Autodesk Fusion 360 part; units mm, degrees
note: some values were not read from the file. Chosen so that the rebuilt part matches the saved one: which face or edge a step refers to. Set by a fixed rule: which sketch regions a step uses.
(part 4 of 4)
sketch "Fingers Bottom" plane through (0, 0, 0) normal (0, 0, 1) x (1, 0, 0) in component "Bottom"
  arc A0 (-85.6137, -27.905) -> (-84, -26.7758) centre (-84.7071, -27.4829) ccw
  arc A1 (-84, -119.2242) -> (-85.6137, -118.095) centre (-84.7071, -118.5171) ccw
  arc A2 (-84, -39.2242) -> (-85.6137, -38.095) centre (-84.7071, -38.5171) ccw
  line L0 (-84, -26.7758) -> (-84, -19.2242)
  arc A3 (-85.6137, -107.905) -> (-84, -106.7758) centre (-84.7071, -107.4829) ccw
  arc A4 (-87.175, -126.7758) -> (-85.5613, -127.905) centre (-86.4679, -127.4829) ccw
  arc A5 (-84, -139.2242) -> (-85.6137, -138.095) centre (-84.7071, -138.5171) ccw
  line L1 (-84, -146.7758) -> (-84, -139.2242)
  line L2 (-85.5613, -107.905) -> (-85.6137, -107.905)
  arc A6 (-87.175, -146.7758) -> (-85.5613, -147.905) centre (-86.4679, -147.4829) ccw
  line L3 (-85.5613, -147.905) -> (-85.6137, -147.905)
  arc A7 (-87.175, -26.7758) -> (-85.5613, -27.905) centre (-86.4679, -27.4829) ccw
  line L4 (-87.175, -119.2242) -> (-87.175, -126.7758)
  line L5 (-85.5613, -127.905) -> (-85.6137, -127.905)
  arc A8 (-85.5613, -18.095) -> (-87.175, -19.2242) centre (-86.4679, -18.5171) ccw
  line L6 (-85.6137, -38.095) -> (-85.5613, -38.095)
  arc A9 (-87.175, -106.7758) -> (-85.5613, -107.905) centre (-86.4679, -107.4829) ccw
  line L7 (-85.6137, -18.095) -> (-85.5613, -18.095)
  line L8 (-85.5613, -27.905) -> (-85.6137, -27.905)
  arc A10 (-85.6137, -127.905) -> (-84, -126.7758) centre (-84.7071, -127.4829) ccw
  line L9 (-85.6137, -118.095) -> (-85.5613, -118.095)
  line L10 (-84, -46.7758) -> (-84, -39.2242)
  arc A11 (-84, -79.2242) -> (-85.6137, -78.095) centre (-84.7071, -78.5171) ccw
  arc A12 (-84, -59.2242) -> (-85.6137, -58.095) centre (-84.7071, -58.5171) ccw
  arc A13 (-85.5613, -58.095) -> (-87.175, -59.2242) centre (-86.4679, -58.5171) ccw
  arc A14 (-87.175, -86.7758) -> (-85.5613, -87.905) centre (-86.4679, -87.4829) ccw
  line L11 (-87.175, -59.2242) -> (-87.175, -66.7758)
  line L12 (0, 0) -> (-240, 0) construction
  line L13 (-85.5613, -47.905) -> (-85.6137, -47.905)
  arc A15 (-87.175, -66.7758) -> (-85.5613, -67.905) centre (-86.4679, -67.4829) ccw
  arc A16 (-87.175, -46.7758) -> (-85.5613, -47.905) centre (-86.4679, -47.4829) ccw
  line L14 (-85.6137, -78.095) -> (-85.5613, -78.095)
  line L15 (-84, -66.7758) -> (-84, -59.2242)
  arc A17 (-85.6137, -47.905) -> (-84, -46.7758) centre (-84.7071, -47.4829) ccw
  line L16 (-87.175, -139.2242) -> (-87.175, -146.7758)
  line L17 (-85.6137, -138.095) -> (-85.5613, -138.095)
  line L18 (-84, -126.7758) -> (-84, -119.2242)
  line L19 (-87.175, -39.2242) -> (-87.175, -46.7758)
  line L20 (-85.6137, -58.095) -> (-85.5613, -58.095)
  arc A18 (-85.6137, -147.905) -> (-84, -146.7758) centre (-84.7071, -147.4829) ccw
  arc A19 (-85.5613, -118.095) -> (-87.175, -119.2242) centre (-86.4679, -118.5171) ccw
  arc A20 (-85.5613, -78.095) -> (-87.175, -79.2242) centre (-86.4679, -78.5171) ccw
  line L21 (-87.175, -99.2242) -> (-87.175, -106.7758)
  arc A21 (-85.5613, -138.095) -> (-87.175, -139.2242) centre (-86.4679, -138.5171) ccw
  line L22 (-87.175, -79.2242) -> (-87.175, -86.7758)
  arc A22 (-84, -99.2242) -> (-85.6137, -98.095) centre (-84.7071, -98.5171) ccw
  line L23 (0, 0) -> (0, -184) construction
  arc A23 (-85.5613, -98.095) -> (-87.175, -99.2242) centre (-86.4679, -98.5171) ccw
  line L24 (-84, -86.7758) -> (-84, -79.2242)
  line L25 (-85.6137, -98.095) -> (-85.5613, -98.095)
  line L26 (-85.5613, -87.905) -> (-85.6137, -87.905)
  arc A24 (-85.6137, -87.905) -> (-84, -86.7758) centre (-84.7071, -87.4829) ccw
  line L27 (0, -184) -> (-240, -184) construction
  line L28 (-240, 0) -> (-240, -184) construction
  line L29 (-85.5613, -67.905) -> (-85.6137, -67.905)
  arc A25 (-85.6137, -67.905) -> (-84, -66.7758) centre (-84.7071, -67.4829) ccw
  arc A26 (-85.5613, -158.095) -> (-87.175, -159.2242) centre (-86.4679, -158.5171) ccw
  arc A27 (-84, -19.2242) -> (-85.6137, -18.095) centre (-84.7071, -18.5171) ccw
  line L30 (-87.175, -19.2242) -> (-87.175, -26.7758)
  arc A28 (-85.6137, -167.905) -> (-84, -166.7758) centre (-84.7071, -167.4829) ccw
  line L31 (-85.6137, -158.095) -> (-85.5613, -158.095)
  line L32 (-84, -166.7758) -> (-84, -159.2242)
  arc A29 (-87.175, -166.7758) -> (-85.5613, -167.905) centre (-86.4679, -167.4829) ccw
  arc A30 (-85.5613, -38.095) -> (-87.175, -39.2242) centre (-86.4679, -38.5171) ccw
  line L33 (-85.5613, -167.905) -> (-85.6137, -167.905)
  line L34 (-87.175, -159.2242) -> (-87.175, -166.7758)
  arc A31 (-84, -159.2242) -> (-85.6137, -158.095) centre (-84.7071, -158.5171) ccw
  line L35 (-84, -106.7758) -> (-84, -99.2242)
  line L36 (-240, -2) -> (0, -2)
  point P0 (0, -184)
  dimension "d1377" = 20
  dimension "d1378" = 20
  dimension "d1379" = 2
  dimension "d1380" = 0.4221
  dimension "d1381" = 9.81
  dimension "d1382" = 2
  dimension "d1383" = 16.095
  dimension "d1384" = 3.175
  dimension "d1385" = 2
  dimension "d1386" = 2
  dimension "d1387" = 0.4221
  dimension "d1388" = 0.4221
  dimension "d1389" = 0.7071
  dimension "d1390" = 0.7071
  dimension "d1391" = 0.7071
  dimension "d1392" = 84
  dimension "d1393" = 0.4221
  dimension "d1395" = 240
  dimension "d1622" = 182
  constraint horizontal L27
  constraint perpendicular L32 L33
  constraint vertical A28.centre A31.centre
  constraint perpendicular L12 L23
  constraint perpendicular L27 L28
  constraint coincident P0 L23.end
  constraint coincident L12.start L23.start
  measures "d1379" diameter of A31
  measures "d1380" distance of A31.centre L31
  measures "d1381" distance of L31 L33
  measures "d1382" diameter of A28
  measures "d1383" distance of L27 L33
  measures "d1384" distance of L32 L34
  measures "d1385" diameter of A26
  measures "d1386" diameter of A29
  measures "d1387" distance of A26.centre L31
  measures "d1388" distance of A29.centre L33
  measures "d1389" distance of A29.centre L34
  measures "d1390" distance of A28.centre L32
  measures "d1391" distance of A26.centre L34
  measures "d1392" distance of L23 L32
  measures "d1393" distance of A28.centre L33
  measures "d1395" distance of L27.end P0
  measures "d1622" distance of L27 L36
sketch "Fingers" plane through (0, 0, 0) normal (0, 0, 1) x (1, 0, 0) in component "Top"
  arc A0 (-85.6137, 16.095) -> (-84, 17.2242) centre (-84.7071, 16.5171) ccw
  arc A1 (-85.6137, 36.095) -> (-84, 37.2242) centre (-84.7071, 36.5171) ccw
  line L0 (-87.175, 44.7758) -> (-87.175, 37.2242)
  arc A2 (-84, 24.7758) -> (-85.6137, 25.905) centre (-84.7071, 25.4829) ccw
  line L1 (-87.175, 24.7758) -> (-87.175, 17.2242)
  line L2 (-87.175, 64.7758) -> (-87.175, 57.2242)
  line L3 (-85.6137, 125.905) -> (-85.5613, 125.905)
  arc A3 (-84, 144.7758) -> (-85.6137, 145.905) centre (-84.7071, 145.4829) ccw
  arc A4 (-85.6137, 156.095) -> (-84, 157.2242) centre (-84.7071, 156.5171) ccw
  arc A5 (-85.5613, 125.905) -> (-87.175, 124.7758) centre (-86.4679, 125.4829) ccw
  line L4 (-87.175, 144.7758) -> (-87.175, 137.2242)
  line L5 (-87.175, 164.7758) -> (-87.175, 157.2242)
  line L6 (-87.175, 104.7758) -> (-87.175, 97.2242)
  line L7 (-85.6137, 145.905) -> (-85.5613, 145.905)
  arc A6 (-85.5613, 105.905) -> (-87.175, 104.7758) centre (-86.4679, 105.4829) ccw
  line L8 (-85.5613, 96.095) -> (-85.6137, 96.095)
  arc A7 (-84, 124.7758) -> (-85.6137, 125.905) centre (-84.7071, 125.4829) ccw
  arc A8 (-87.175, 137.2242) -> (-85.5613, 136.095) centre (-86.4679, 136.5171) ccw
  line L9 (-85.5613, 116.095) -> (-85.6137, 116.095)
  arc A9 (-84, 84.7758) -> (-85.6137, 85.905) centre (-84.7071, 85.4829) ccw
  line L10 (-84, 157.2242) -> (-84, 164.7758)
  line L11 (-85.5613, 156.095) -> (-85.6137, 156.095)
  line L12 (-84, 137.2242) -> (-84, 144.7758)
  arc A10 (-85.6137, 116.095) -> (-84, 117.2242) centre (-84.7071, 116.5171) ccw
  line L13 (-85.6137, 165.905) -> (-85.5613, 165.905)
  arc A11 (-84, 164.7758) -> (-85.6137, 165.905) centre (-84.7071, 165.4829) ccw
  arc A12 (-87.175, 157.2242) -> (-85.5613, 156.095) centre (-86.4679, 156.5171) ccw
  arc A13 (-85.5613, 165.905) -> (-87.175, 164.7758) centre (-86.4679, 165.4829) ccw
  line L14 (-85.6137, 85.905) -> (-85.5613, 85.905)
  arc A14 (-87.175, 117.2242) -> (-85.5613, 116.095) centre (-86.4679, 116.5171) ccw
  arc A15 (-85.6137, 96.095) -> (-84, 97.2242) centre (-84.7071, 96.5171) ccw
  arc A16 (-85.5613, 145.905) -> (-87.175, 144.7758) centre (-86.4679, 145.4829) ccw
  arc A17 (-85.5613, 85.905) -> (-87.175, 84.7758) centre (-86.4679, 85.4829) ccw
  arc A18 (-87.175, 97.2242) -> (-85.5613, 96.095) centre (-86.4679, 96.5171) ccw
  arc A19 (-87.175, 37.2242) -> (-85.5613, 36.095) centre (-86.4679, 36.5171) ccw
  arc A20 (-84, 44.7758) -> (-85.6137, 45.905) centre (-84.7071, 45.4829) ccw
  line L15 (0, 0) -> (-240, 0) construction
  line L16 (-85.5613, 16.095) -> (-85.6137, 16.095)
  arc A21 (-85.5613, 25.905) -> (-87.175, 24.7758) centre (-86.4679, 25.4829) ccw
  line L17 (-85.6137, 65.905) -> (-85.5613, 65.905)
  line L18 (-84, 37.2242) -> (-84, 44.7758)
  line L19 (-85.6137, 45.905) -> (-85.5613, 45.905)
  arc A22 (-87.175, 17.2242) -> (-85.5613, 16.095) centre (-86.4679, 16.5171) ccw
  arc A23 (-87.175, 57.2242) -> (-85.5613, 56.095) centre (-86.4679, 56.5171) ccw
  line L20 (-85.5613, 36.095) -> (-85.6137, 36.095)
  arc A24 (-84, 64.7758) -> (-85.6137, 65.905) centre (-84.7071, 65.4829) ccw
  line L21 (0, 182) -> (-240, 182) construction
  arc A25 (-85.5613, 45.905) -> (-87.175, 44.7758) centre (-86.4679, 45.4829) ccw
  arc A26 (-85.5613, 65.905) -> (-87.175, 64.7758) centre (-86.4679, 65.4829) ccw
  line L22 (-87.175, 84.7758) -> (-87.175, 77.2242)
  line L23 (-84, 57.2242) -> (-84, 64.7758)
  arc A27 (-85.6137, 136.095) -> (-84, 137.2242) centre (-84.7071, 136.5171) ccw
  line L24 (-84, 17.2242) -> (-84, 24.7758)
  line L25 (-85.6137, 25.905) -> (-85.5613, 25.905)
  arc A28 (-85.6137, 56.095) -> (-84, 57.2242) centre (-84.7071, 56.5171) ccw
  line L26 (-240, 182) -> (-240, 0) construction
  line L27 (0, 182) -> (0, 0) construction
  line L28 (-85.5613, 56.095) -> (-85.6137, 56.095)
  line L29 (-84, 77.2242) -> (-84, 84.7758)
  line L30 (-84, 117.2242) -> (-84, 124.7758)
  arc A29 (-87.175, 77.2242) -> (-85.5613, 76.095) centre (-86.4679, 76.5171) ccw
  line L31 (-85.6137, 105.905) -> (-85.5613, 105.905)
  arc A30 (-84, 104.7758) -> (-85.6137, 105.905) centre (-84.7071, 105.4829) ccw
  line L32 (-84, 97.2242) -> (-84, 104.7758)
  line L33 (-87.175, 124.7758) -> (-87.175, 117.2242)
  line L34 (-85.5613, 76.095) -> (-85.6137, 76.095)
  arc A31 (-85.6137, 76.095) -> (-84, 77.2242) centre (-84.7071, 76.5171) ccw
  line L35 (-85.5613, 136.095) -> (-85.6137, 136.095)
  dimension "d1479" = 20
  dimension "d1480" = 20
  dimension "d1481" = 2
  dimension "d1482" = 0.4221
  dimension "d1483" = 9.81
  dimension "d1484" = 2
  dimension "d1485" = 16.095
  dimension "d1486" = 3.175
  dimension "d1487" = 2
  dimension "d1488" = 2
  dimension "d1489" = 0.4221
  dimension "d1490" = 0.4221
  dimension "d1491" = 0.7071
  dimension "d1492" = 0.7071
  dimension "d1493" = 0.7071
  dimension "d1494" = 84
  dimension "d1495" = 0.4221
  dimension "d1496" = 182
  dimension "d1497" = 240
  constraint horizontal L15
  constraint perpendicular L16 L24
  constraint vertical A2.centre A0.centre
  constraint perpendicular L21 L27
  constraint perpendicular L15 L26
  constraint coincident L15.start L27.end
  measures "d1481" diameter of A2
  measures "d1482" distance of A2.centre L25
  measures "d1483" distance of L16 L25
  measures "d1484" diameter of A0
  measures "d1485" distance of L15 L16
  measures "d1486" distance of L1 L24
  measures "d1487" diameter of A21
  measures "d1488" diameter of A22
  measures "d1489" distance of A21.centre L25
  measures "d1490" distance of A22.centre L16
  measures "d1491" distance of A22.centre L1
  measures "d1492" distance of A0.centre L24
  measures "d1493" distance of A21.centre L1
  measures "d1494" distance of L24 L27
  measures "d1495" distance of A0.centre L16
  measures "d1496" distance of L15.start L21.start
  measures "d1497" distance of L15.end L15.start
sketch "Projection" plane through (0, 0, 0) normal (0, 0, 1) x (1, 0, 0) in component "Brace"
  line L0 (3.175, 14.7758) -> (3.175, 0)
  line L1 (3.175, 0) -> (15.095, 0)
  line L2 (15.095, 0) -> (15.095, 1.5613)
  arc A0 (16.2242, 3.175) -> (15.095, 1.5613) centre (15.5171, 2.4679) ccw
  line L3 (16.2242, 3.175) -> (23.7758, 3.175)
  arc A1 (24.905, 1.5613) -> (23.7758, 3.175) centre (24.4829, 2.4679) ccw
  line L4 (24.905, 1.5613) -> (24.905, 0)
  line L5 (24.905, 0) -> (35.095, 0)
  line L6 (35.095, 0) -> (35.095, 1.5613)
  arc A2 (36.2242, 3.175) -> (35.095, 1.5613) centre (35.5171, 2.4679) ccw
  line L7 (36.2242, 3.175) -> (43.7758, 3.175)
  arc A3 (44.905, 1.5613) -> (43.7758, 3.175) centre (44.4829, 2.4679) ccw
  line L8 (44.905, 1.5613) -> (44.905, 0)
  line L9 (44.905, 0) -> (56.825, 0)
  line L10 (56.825, 0) -> (56.825, 14.7758)
  arc A4 (58.4387, 15.905) -> (56.825, 14.7758) centre (57.5321, 15.4829) ccw
  line L11 (58.4387, 15.905) -> (60, 15.905)
  line L12 (60, 15.905) -> (60, 26.095)
  line L13 (60, 26.095) -> (58.4387, 26.095)
  arc A5 (56.825, 27.2242) -> (58.4387, 26.095) centre (57.5321, 26.5171) ccw
  line L14 (56.825, 27.2242) -> (56.825, 34.7758)
  arc A6 (58.4387, 35.905) -> (56.825, 34.7758) centre (57.5321, 35.4829) ccw
  line L15 (58.4387, 35.905) -> (60, 35.905)
  line L16 (60, 35.905) -> (60, 46.095)
  line L17 (60, 46.095) -> (58.4387, 46.095)
  arc A7 (56.825, 47.2242) -> (58.4387, 46.095) centre (57.5321, 46.5171) ccw
  line L18 (56.825, 47.2242) -> (56.825, 54.7758)
  arc A8 (58.4387, 55.905) -> (56.825, 54.7758) centre (57.5321, 55.4829) ccw
  line L19 (58.4387, 55.905) -> (60, 55.905)
  line L20 (60, 55.905) -> (60, 66.095)
  line L21 (60, 66.095) -> (58.4387, 66.095)
  arc A9 (56.825, 67.2242) -> (58.4387, 66.095) centre (57.5321, 66.5171) ccw
  line L22 (56.825, 67.2242) -> (56.825, 74.7758)
  arc A10 (58.4387, 75.905) -> (56.825, 74.7758) centre (57.5321, 75.4829) ccw
  line L23 (58.4387, 75.905) -> (60, 75.905)
  line L24 (60, 75.905) -> (60, 86.095)
  line L25 (60, 86.095) -> (58.4387, 86.095)
  arc A11 (56.825, 87.2242) -> (58.4387, 86.095) centre (57.5321, 86.5171) ccw
  line L26 (56.825, 87.2242) -> (56.825, 94.7758)
  arc A12 (58.4387, 95.905) -> (56.825, 94.7758) centre (57.5321, 95.4829) ccw
  line L27 (58.4387, 95.905) -> (60, 95.905)
  line L28 (60, 95.905) -> (60, 106.095)
  line L29 (60, 106.095) -> (58.4387, 106.095)
  arc A13 (56.825, 107.2242) -> (58.4387, 106.095) centre (57.5321, 106.5171) ccw
  line L30 (56.825, 107.2242) -> (56.825, 114.7758)
  arc A14 (58.4387, 115.905) -> (56.825, 114.7758) centre (57.5321, 115.4829) ccw
  line L31 (58.4387, 115.905) -> (60, 115.905)
  line L32 (60, 115.905) -> (60, 126.095)
  line L33 (60, 126.095) -> (58.4387, 126.095)
  arc A15 (56.825, 127.2242) -> (58.4387, 126.095) centre (57.5321, 126.5171) ccw
  line L34 (56.825, 127.2242) -> (56.825, 134.7758)
  arc A16 (58.4387, 135.905) -> (56.825, 134.7758) centre (57.5321, 135.4829) ccw
  line L35 (58.4387, 135.905) -> (60, 135.905)
  line L36 (60, 135.905) -> (60, 146.095)
  line L37 (60, 146.095) -> (58.4387, 146.095)
  arc A17 (56.825, 147.2242) -> (58.4387, 146.095) centre (57.5321, 146.5171) ccw
  line L38 (56.825, 147.2242) -> (56.825, 154.7758)
  arc A18 (58.4387, 155.905) -> (56.825, 154.7758) centre (57.5321, 155.4829) ccw
  line L39 (58.4387, 155.905) -> (60, 155.905)
  line L40 (60, 155.905) -> (60, 166.095)
  line L41 (60, 166.095) -> (58.4387, 166.095)
  arc A19 (56.825, 167.2242) -> (58.4387, 166.095) centre (57.5321, 166.5171) ccw
  line L42 (56.825, 167.2242) -> (56.825, 182)
  line L43 (56.825, 182) -> (44.905, 182)
  line L44 (44.905, 182) -> (44.905, 180.4387)
  arc A20 (43.7758, 178.825) -> (44.905, 180.4387) centre (44.4829, 179.5321) ccw
  line L45 (43.7758, 178.825) -> (36.2242, 178.825)
  arc A21 (35.095, 180.4387) -> (36.2242, 178.825) centre (35.5171, 179.5321) ccw
  line L46 (35.095, 180.4387) -> (35.095, 182)
  line L47 (35.095, 182) -> (24.905, 182)
  line L48 (24.905, 182) -> (24.905, 180.4387)
  arc A22 (23.7758, 178.825) -> (24.905, 180.4387) centre (24.4829, 179.5321) ccw
  line L49 (23.7758, 178.825) -> (16.2242, 178.825)
  arc A23 (15.095, 180.4387) -> (16.2242, 178.825) centre (15.5171, 179.5321) ccw
  line L50 (15.095, 180.4387) -> (15.095, 182)
  line L51 (15.095, 182) -> (3.175, 182)
  line L52 (3.175, 182) -> (3.175, 167.2242)
  arc A24 (1.5613, 166.095) -> (3.175, 167.2242) centre (2.4679, 166.5171) ccw
  line L53 (1.5613, 166.095) -> (0, 166.095)
  line L54 (0, 166.095) -> (0, 155.905)
  line L55 (0, 155.905) -> (1.5613, 155.905)
  arc A25 (3.175, 154.7758) -> (1.5613, 155.905) centre (2.4679, 155.4829) ccw
  line L56 (3.175, 154.7758) -> (3.175, 147.2242)
  arc A26 (1.5613, 146.095) -> (3.175, 147.2242) centre (2.4679, 146.5171) ccw
  line L57 (1.5613, 146.095) -> (0, 146.095)
  line L58 (0, 146.095) -> (0, 135.905)
  line L59 (0, 135.905) -> (1.5613, 135.905)
  arc A27 (3.175, 134.7758) -> (1.5613, 135.905) centre (2.4679, 135.4829) ccw
  line L60 (3.175, 134.7758) -> (3.175, 127.2242)
  arc A28 (1.5613, 126.095) -> (3.175, 127.2242) centre (2.4679, 126.5171) ccw
  line L61 (1.5613, 126.095) -> (0, 126.095)
  line L62 (0, 126.095) -> (0, 115.905)
  line L63 (0, 115.905) -> (1.5613, 115.905)
  arc A29 (3.175, 114.7758) -> (1.5613, 115.905) centre (2.4679, 115.4829) ccw
  line L64 (3.175, 114.7758) -> (3.175, 107.2242)
  arc A30 (1.5613, 106.095) -> (3.175, 107.2242) centre (2.4679, 106.5171) ccw
  line L65 (1.5613, 106.095) -> (0, 106.095)
  line L66 (0, 106.095) -> (0, 95.905)
  line L67 (0, 95.905) -> (1.5613, 95.905)
  arc A31 (3.175, 94.7758) -> (1.5613, 95.905) centre (2.4679, 95.4829) ccw
  line L68 (3.175, 94.7758) -> (3.175, 87.2242)
  arc A32 (1.5613, 86.095) -> (3.175, 87.2242) centre (2.4679, 86.5171) ccw
  line L69 (1.5613, 86.095) -> (0, 86.095)
  line L70 (0, 86.095) -> (0, 75.905)
  line L71 (0, 75.905) -> (1.5613, 75.905)
  arc A33 (3.175, 74.7758) -> (1.5613, 75.905) centre (2.4679, 75.4829) ccw
  line L72 (3.175, 74.7758) -> (3.175, 67.2242)
  arc A34 (1.5613, 66.095) -> (3.175, 67.2242) centre (2.4679, 66.5171) ccw
  line L73 (1.5613, 66.095) -> (0, 66.095)
  line L74 (0, 66.095) -> (0, 55.905)
  line L75 (0, 55.905) -> (1.5613, 55.905)
  arc A35 (3.175, 54.7758) -> (1.5613, 55.905) centre (2.4679, 55.4829) ccw
  line L76 (3.175, 54.7758) -> (3.175, 47.2242)
  arc A36 (1.5613, 46.095) -> (3.175, 47.2242) centre (2.4679, 46.5171) ccw
  line L77 (1.5613, 46.095) -> (0, 46.095)
  line L78 (0, 46.095) -> (0, 35.905)
  line L79 (0, 35.905) -> (1.5613, 35.905)
  arc A37 (3.175, 34.7758) -> (1.5613, 35.905) centre (2.4679, 35.4829) ccw
  line L80 (3.175, 34.7758) -> (3.175, 27.2242)
  arc A38 (1.5613, 26.095) -> (3.175, 27.2242) centre (2.4679, 26.5171) ccw
  line L81 (1.5613, 26.095) -> (0, 26.095)
  line L82 (0, 26.095) -> (0, 15.905)
  line L83 (0, 15.905) -> (1.5613, 15.905)
  arc A39 (3.175, 14.7758) -> (1.5613, 15.905) centre (2.4679, 15.4829) ccw
sketch "pHSUpport" plane through (0, 0, 0) normal (0, 0, 1) x (1, 0, 0)
  line L0 (-126.3121, 423.4789) -> (-0.0021, 423.4789)
  line L1 (-0.0021, 423.4789) -> (-0.0021, 307.4298)
  line L2 (-63.1571, 307.4298) -> (-126.3121, 307.4298)
  line L3 (-126.3121, 307.4298) -> (-126.3121, 423.4789)
  circle A0 centre (-95.0428, 331.8598) radius 15
  line L4 (-63.1571, 307.4298) -> (-63.1571, 368.1283)
  line L5 (-63.1571, 368.1283) -> (-0.0021, 368.1283)
  dimension "d1660" = 30
  constraint horizontal L0
  constraint vertical L1
  constraint horizontal L2
  constraint vertical L3
  constraint perpendicular L2 L4
  constraint coincident L1 L5.end
  constraint perpendicular L1 L5
  measures "d1660" diameter of A0
sketch "Sketch1" plane through (0, 0, 0) normal (0, 0, 1) x (1, 0, 0) in component "Peristaltic Pump Support"
  circle A0 centre (53.5964, 47.8456) radius 1.5
  circle A1 centre (22.5964, 47.8456) radius 1.5
  line L0 (55.0964, 58.3456) -> (55.0964, 6.3456) construction
  circle A2 centre (38.0964, 32.3456) radius 15
  line L1 (21.0964, 58.3456) -> (55.0964, 58.3456) construction
  circle A3 centre (38.0964, 56.8456) radius 1.5
  line L2 (55.0964, 6.3456) -> (21.0964, 6.3456) construction
  circle A4 centre (22.5964, 16.8456) radius 1.5
  line L3 (21.0964, 6.3456) -> (21.0964, 58.3456) construction
  circle A5 centre (53.5964, 16.8456) radius 1.5
  circle A6 centre (38.0964, 7.8456) radius 1.5
  point P0 (38.0964, 6.3456)
  point P1 (21.0964, 32.3456)
  point P2 (38.0964, 58.3456)
  dimension "d1669" = 31
  dimension "d1670" = -31
  dimension "d1673" = 0
  dimension "d1674" = 49
  dimension "d1675" = 30
  dimension "d1676" = 15.5
  dimension "d1677" = 34
  dimension "d1678" = 52
  dimension "d1679" = 15.5
  dimension "d1680" = 3
  dimension "d1681" = 3
  constraint horizontal L1
  constraint perpendicular L0 L1
  constraint parallel L1 L2
  constraint parallel L0 L3
  constraint midpoint P1 L3
  constraint horizontal P1 A2.centre
  constraint midpoint P0 L2
  constraint vertical P0 A2.centre
  constraint tangent L2 A6
  constraint midpoint P2 L1
  constraint vertical P2 A3.centre
  measures "d1675" diameter of A2
  measures "d1676" vertical distance of A1.centre A2.centre
  measures "d1677" distance of L0.start L1.start
  measures "d1678" distance of L1.start L2.end
  measures "d1679" horizontal distance of A1.centre A2.centre
  measures "d1680" diameter of A6
  measures "d1681" diameter of A1
equation "fingerWidth = 10 mm"
equation "length = 240 mm"
equation "thickness = 3.175 mm"
equation "height = 60 mm"
equation "d12 = holeWidth"
equation "d13 = thickness"
equation "d14 = thickness"
equation "d15 = thickness"
equation "d21 = lengthCuts"
equation "d23 = -2 * fingerWidth"
equation "toolDiameter = 2 mm"
equation "d34 = toolDiameter"
equation "d36 = boneCenterToHoleSide"
equation "d37 = boneCenterToHoleBig"
equation "d38 = boneCenterToHoleSide"
equation "boneCenterToHoleBig = toolDiameter / 2 / sqrt(2) - 0 * kerf" comment "Best: 2.001 -2*kerf, 0.1;;;Best: 2.001 no kerf and 0.1   OLD+6 kerf at 2.001 Diam and .1 mm"
equation "tempLengthPieces = ceil(( ( floor(( length - 2 * thickness ) / fingerWidth) - 2 ) - ( ( floor(( length - 2 * thickness ) / fingerWidth) - 2 ) % 2 - 1 ) ))"
equation "lengthCuts = ceil(tempLengthPieces / 2)"
equation "shoulderToothLength = ( length - fingerWidth * tempLengthPieces ) / 2 - kerf"
equation "depth = 182 mm"
equation "tempDepthPieces = ceil(( ( floor(( depth - 2 * thickness ) / fingerWidth) - 2 ) - ( ( floor(( depth - 2 * thickness ) / fingerWidth) - 2 ) % 2 - 1 ) ))"
equation "depthCuts = ceil(tempDepthPieces / 2)"
equation "shoulderToothDepth = ( depth - fingerWidth * tempDepthPieces ) / 2 - kerf"
equation "d48 = toolDiameter"
equation "d49 = boneCenterToHoleSide"
equation "d50 = shoulderToothDepth"
equation "d51 = thickness"
equation "d52 = boneCenterToHoleSide"
equation "d54 = boneCenterToHoleBig"
equation "d55 = holeWidth"
equation "d56 = depthCuts"
equation "d58 = 2 * fingerWidth"
equation "d80 = depth"
equation "d82 = holeWidth"
equation "d85 = height"
equation "d86 = toolDiameter"
equation "d87 = boneCenterToHoleSide"
equation "d88 = boneCenterToHoleBig"
equation "d89 = boneCenterToHoleSide"
equation "d98 = toolDiameter"
equation "d99 = shouderHoleDepth"
equation "d100 = thickness"
equation "tempHeightPieces = ceil(( ( floor(( height - 2 * thickness ) / fingerWidth) - 2 ) - ( ( floor(( height - 2 * thickness ) / fingerWidth) - 2 ) % 2 - 1 ) ))"
equation "heightCuts = ceil(tempHeightPieces / 2)"
equation "sholderToothHeight = ( height - fingerWidth * tempHeightPieces ) / 2 - kerf"
equation "d104 = thickness"
equation "d105 = holeWidth"
equation "d113 = toolDiameter"
equation "d114 = boneCenterToHoleBig"
equation "d115 = boneCenterToHoleSide"
equation "d116 = toolDiameter"
equation "d117 = boneCenterToHoleSide"
equation "d119 = boneCenterToHoleSide"
equation "d122 = sholderToothHeight"
equation "d126 = thickness"
equation "d128 = heightCuts"
equation "d130 = -2 * fingerWidth"
equation "d132 = depthCuts - 2"
equation "d134 = -2 * fingerWidth"
equation "d140 = height"
equation "d141 = holeWidth"
equation "d142 = thickness"
equation "d143 = thickness"
equation "d144 = length"
equation "d145 = toolDiameter"
equation "d146 = boneCenterToHoleSide"
equation "d147 = boneCenterToHoleBig"
equation "d148 = boneCenterToHoleSide"
equation "d149 = shoulderHoleHeight"
equation "d150 = thickness"
equation "d151 = thickness"
equation "d152 = holeWidth"
equation "d154 = toolDiameter"
equation "d155 = boneCenterToHoleBig"
equation "d156 = boneCenterToHoleSide"
equation "d157 = toolDiameter"
equation "d159 = boneCenterToHoleSide"
equation "d160 = thickness"
equation "d163 = toolDiameter"
equation "d164 = boneCenterToHoleSide"
equation "d169 = thickness"
equation "d171 = fingerWidth - 2 * kerf"
equation "d172 = lengthCuts - 1"
equation "d174 = -2 * fingerWidth"
equation "d178 = heightCuts"
equation "d180 = -2 * fingerWidth"
equation "d182 = boneCenterToHoleSide"
equation "d183 = thickness"
equation "d184 = toolDiameter"
equation "d185 = toolDiameter"
equation "d186 = boneCenterToHoleSide"
equation "d187 = boneCenterToHoleSide"
equation "d189 = shoulderToothLength"
equation "d191 = shoulderHoleLength"
equation "d192 = fingerWidth - 2 * kerf"
equation "d193 = shoulderHoleLength"
equation "kerf = -0.095 mm"
equation "holeWidth = fingerWidth + 2 * kerf"
equation "shoulderHoleLength = shoulderToothLength + 2 * kerf"
equation "shouderHoleDepth = shoulderToothDepth + 2 * kerf"
equation "shoulderHoleHeight = sholderToothHeight + 2 * kerf"
equation "d354 = fingerWidth - 2 * kerf"
equation "assembleScrewDiam = 2.1 mm"
equation "assembleScrewDistance = 6 mm"
equation "assembleAvoidCollisionDistance = 1 mm"
equation "coolingHoleDistance = 8 mm"
equation "boneCornerToCenterPack = -3 * kerf"
equation "boneCenterToHoleSide = boneCenterToHoleBig - boneCornerToCenterPack"
equation "d416 = boneCenterToHoleSide"
equation "d417 = shouderHoleDepth"
equation "d418 = shoulderHoleHeight"
equation "d442 = thickness"
equation "d473 = length"
equation "d474 = toolDiameter"
equation "d475 = depth"
equation "d476 = toolDiameter"
equation "d479 = -toolDiameter / 2"
equation "d282 = platformGrommetMountDiameter"
equation "d289 = pcbMountHoles"
equation "d422 = length"
equation "d423 = depth"
equation "d463 = toolDiameter + 0.1 mm"
equation "d843 = toolDiameter"
equation "d523 = depth"
equation "pumpLength = 52 mm"
equation "pumpCircleDiam = 30 mm"
equation "pumpHeight = 34 mm"
equation "sensorWireDistance = 10 mm"
equation "sensorWireDiam = 3.5 mm"
equation "pumpScrewDiam = 3 mm"
equation "d846 = hangerWireDiameter"
equation "d910 = depth"
equation "d911 = height"
equation "d930 = sensorWireDiam"
equation "d1194 = depth / 2"
equation "d993 = length + toolDiameter"
equation "d502 = length"
equation "d503 = height"
equation "d870 = ventDiameter"
equation "d1047 = toolDiameter"
equation "d1048 = 3 * toolDiameter"
equation "d492 = length"
equation "d493 = height"
equation "d1106 = toolDiameter"
equation "d1136 = depth"
equation "d1137 = height"
equation "d1162 = -topPillowHoleDistance"
equation "d1163 = length"
equation "d1164 = depth"
equation "d1173 = ventDiameter"
equation "d1177 = ( depth - topPillowHoleDistance ) / 2"
equation "d1086 = toolDiameter"
equation "d1087 = boneCenterToHoleSide"
equation "d1091 = fingerWidth - 2 * kerf"
equation "d1094 = toolDiameter"
equation "d1109 = boneCenterToHoleSide"
equation "d1113 = toolDiameter"
equation "d1116 = thickness"
equation "d1117 = boneCenterToHoleBig"
equation "d1221 = toolDiameter"
equation "d1222 = toolDiameter"
equation "d1223 = toolDiameter"
equation "d1224 = toolDiameter"
equation "d1225 = toolDiameter"
equation "d1227 = boneCenterToHoleBig"
equation "d1228 = boneCenterToHoleBig"
equation "d1229 = boneCenterToHoleSide"
equation "d1230 = boneCenterToHoleSide"
equation "d1232 = boneCenterToHoleSide"
equation "d1233 = boneCenterToHoleSide"
equation "d1235 = boneCenterToHoleBig"
equation "d1236 = boneCenterToHoleBig"
equation "d1178 = boneCenterToHoleBig"
equation "d1323 = length"
equation "d1376 = depthCuts"
equation "d1378 = 2 * fingerWidth"
equation "d1379 = toolDiameter"
equation "d1380 = boneCenterToHoleSide"
equation "d1381 = holeWidth"
equation "d1382 = toolDiameter"
equation "d1383 = shoulderToothDepth"
equation "d1384 = thickness"
equation "d1385 = toolDiameter"
equation "d1386 = toolDiameter"
equation "d1387 = boneCenterToHoleSide"
equation "d1388 = boneCenterToHoleSide"
equation "d1389 = boneCenterToHoleBig"
equation "d1390 = boneCenterToHoleBig"
equation "d1391 = boneCenterToHoleBig"
equation "d1393 = boneCenterToHoleSide"
equation "d1395 = length"
equation "d1399 = toolDiameter"
equation "d1400 = toolDiameter"
equation "d1401 = length + toolDiameter"
equation "d1404 = toolDiameter"
equation "d1405 = boneCenterToHoleSide"
equation "d1406 = fingerWidth - 2 * kerf"
equation "d1407 = toolDiameter"
equation "d1408 = boneCenterToHoleSide"
equation "d1409 = toolDiameter"
equation "d1412 = boneCenterToHoleBig"
equation "d1413 = toolDiameter"
equation "d1414 = toolDiameter"
equation "d1415 = toolDiameter"
equation "d1416 = toolDiameter"
equation "d1417 = toolDiameter"
equation "d1418 = boneCenterToHoleBig"
equation "d1419 = boneCenterToHoleBig"
equation "d1420 = boneCenterToHoleSide"
equation "d1421 = boneCenterToHoleSide"
equation "d1423 = boneCenterToHoleSide"
equation "d1424 = boneCenterToHoleSide"
equation "d1425 = boneCenterToHoleBig"
equation "d1426 = boneCenterToHoleBig"
equation "d1427 = boneCenterToHoleBig"
equation "d1428 = length"
equation "d1431 = shoulderHoleHeight"
equation "d1433 = holeWidth"
equation "d1436 = toolDiameter"
equation "d1437 = shoulderHoleHeight"
equation "d1440 = 3 * toolDiameter"
equation "d1441 = boneCenterToHoleSide"
equation "d1442 = boneCenterToHoleSide"
equation "d1443 = boneCenterToHoleBig"
equation "d1444 = boneCenterToHoleBig"
equation "d1446 = thickness"
equation "d1447 = thickness"
equation "d1451 = thickness"
equation "d1452 = height"
equation "d1453 = thickness"
equation "d1454 = thickness"
equation "d1456 = boneCenterToHoleSide"
equation "d1457 = boneCenterToHoleSide"
equation "d1460 = height"
equation "d1461 = toolDiameter"
equation "d1462 = thickness"
equation "d1463 = thickness"
equation "d1466 = holeWidth"
equation "d1468 = shoulderHoleHeight"
equation "d1469 = shoulderHoleHeight"
equation "d1472 = boneCenterToHoleBig"
equation "d1473 = boneCenterToHoleBig"
equation "pcbMountHoles = 2 mm"
equation "d1481 = toolDiameter"
equation "d1482 = boneCenterToHoleSide"
equation "d1483 = holeWidth"
equation "d1484 = toolDiameter"
equation "d1485 = shoulderToothDepth"
equation "d1486 = thickness"
equation "d1487 = toolDiameter"
equation "d1488 = toolDiameter"
equation "d1489 = boneCenterToHoleSide"
equation "d1490 = boneCenterToHoleSide"
equation "d1491 = boneCenterToHoleBig"
equation "d1492 = boneCenterToHoleBig"
equation "d1493 = boneCenterToHoleBig"
equation "d1495 = boneCenterToHoleSide"
equation "d1496 = depth"
equation "d1497 = length"
equation "d1515 = platformGrommetMountDiameter"
equation "d1516 = platformGrommetMountDiameter"
equation "d1517 = platformGrommetMountDiameter"
equation "d1518 = platformGrommetMountDiameter"
equation "ventDiameter = 3 mm"
equation "d1542 = height"
equation "platformGrommetMountDiameter = 3.5 mm"
equation "d1557 = platformGrommetMountDiameter"
equation "d1558 = platformGrommetMountDiameter"
equation "d1559 = platformGrommetMountDiameter"
equation "d1560 = platformGrommetMountDiameter"
equation "d1561 = sensorWireDiam"
equation "d1567 = 11 mm + thickness"
equation "d1571 = toolDiameter"
equation "d1573 = toolDiameter"
equation "d1574 = boneCenterToHoleBig"
equation "d1575 = boneCenterToHoleBig"
equation "d1576 = boneCenterToHoleSide"
equation "d1577 = boneCenterToHoleSide"
equation "d1578 = toolDiameter"
equation "d1579 = toolDiameter"
equation "d1580 = boneCenterToHoleSide"
equation "d1581 = boneCenterToHoleSide"
equation "d1582 = boneCenterToHoleBig"
equation "d1583 = boneCenterToHoleBig"
equation "d1584 = toolDiameter"
equation "d1585 = toolDiameter"
equation "d1586 = boneCenterToHoleBig"
equation "d1587 = boneCenterToHoleSide"
equation "d1588 = boneCenterToHoleSide"
equation "d1589 = boneCenterToHoleBig"
equation "d1590 = toolDiameter"
equation "d1591 = toolDiameter"
equation "d1592 = boneCenterToHoleBig"
equation "d1593 = boneCenterToHoleBig"
equation "d1594 = boneCenterToHoleSide"
equation "d1595 = boneCenterToHoleSide"
equation "d1609 = thickness"
equation "d1618 = thickness"
equation "d1621 = depth + toolDiameter"
equation "d1622 = depth"
equation "d1640 = 48 mm + thickness - ( 49 / 2 ) * 1 mm"
equation "hangerWireDiameter = 2 mm"
equation "topPillowHoleDistance = 22 mm"
equation "d1675 = pumpCircleDiam"
equation "d1677 = pumpHeight"
equation "d1678 = pumpLength"
equation "d1679 = ( pumpHeight - pumpScrewDiam ) / 2"
equation "d1680 = pumpScrewDiam"
equation "d1696 = ventDiameter"
equation "d1705 = ventDiameter"
equation "d1716 = thickness"
equation "d1722 = toolDiameter"
equation "d1726 = toolDiameter + 0.001 mm"
equation "d1748 = pumpScrewDiam"
equation "d1754 = ( 41 / 2 ) * 1 mm + thickness + 2 mm"
equation "d1757 = -41 mm - 6 mm"
equation "d1766 = pumpScrewDiam"
equation "d1783 = 360.0 °"
named bodies: "Side", "Box Front", "Box Top", "Box Right", "Front (1)", "Box Right Side (1)", "Box Bottom (1)", "Box Bottom", "Box  Left", "Box Back", "Brace", "Platform", "Box Top (1)"
